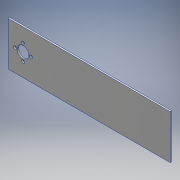
# Autodesk Inventor part: snap
Saved by Autodesk Inventor 2016 (Build 200138000, 138)
## iProperties
Created: 2016-06-28
Part Number: snap
Material: アルミニウム 6061
Document SubType Name: Modeling
Designer: 宏太
Density: 2.7 g/cm^3
Appearance: アルミニウム - フラット
Mass: 253.66 g
Surface Area: 284.714 cm^2
Volume: 93.9482 cm^3
Author: 宏太
Autodesk Inventor part; units mm, degrees
ref_plane "YZ Plane" through (0, 0, 0) normal (1, 0, 0) x (0, 1, 0)
ref_plane "XZ Plane" through (0, 0, 0) normal (0, 1, 0) x (-1, 0, 0)
ref_plane "XY Plane" through (0, 0, 0) normal (0, 0, 1) x (1, 0, 0)
sketch "スケッチ1" plane through (0, 0, 0) normal (0, 1, 0) x (-1, 0, 0)
  line L0 (-110, -30) -> (110, -30)
  line L1 (110, -30) -> (110, 30)
  line L2 (110, 30) -> (-110, 30)
  line L3 (-110, 30) -> (-110, -30)
  line L4 (-110, -30) -> (110, 30) construction
  line L5 (110, -30) -> (-110, 30) construction
  point P0 (0, 0)
  dimension "d0" = 220
  dimension "d1" = 60
  constraints: 12 end point, 2 midpoint, 2 parallel, 1 horizontal, 1 perpendicular
  measures "d0" distance of L2.end L1.end
  measures "d1" distance of L1.end L0.end
extrude "押し出し1" add sketch "スケッチ1" along normal blind 2
sketch "スケッチ2" plane through (0, 2, 0) normal (0, 1, 0) x (1, 0, 0)
  circle A0 centre (-90, 0) radius 8
  circle A1 centre (-101, 0) radius 2.1
  circle A2 centre (-90, 11) radius 2.1
  circle A3 centre (-79, 0) radius 2.1
  circle A4 centre (-90, -11) radius 2.1
  point P0 (0, 0)
  dimension "d4" = 16
  dimension "d5" = 90
  dimension "d7" = 4.2
  dimension "d8" = 4.2
  dimension "d9" = 4.2
  dimension "d10" = 4.2
  dimension "d13" = 11
  dimension "d14" = 11
  dimension "d15" = 11
  dimension "d16" = 11
  constraints: 5 centre point
  measures "d4" diameter of A0
  measures "d5" distance of point (0, 0) A0.centre
  measures "d7" diameter of A1
  measures "d8" diameter of A2
  measures "d9" diameter of A3
  measures "d10" diameter of A4
  measures "d13" distance of A0.centre A1.centre
  measures "d14" distance of A4.centre A0.centre
  measures "d15" distance of A2.centre A0.centre
  measures "d16" distance of A0.centre A3.centre
extrude "押し出し2" cut sketch "スケッチ2" against normal blind 8
